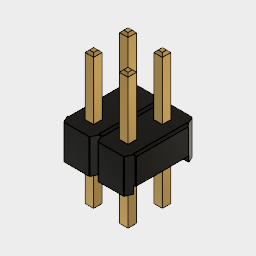
Pin+Header+2x2+TH+Pitch+2 (Autodesk Fusion 360 design; units mm, degrees)
Autodesk Fusion 360 part; units mm, degrees
note: some values were not read from the file. Chosen so that the rebuilt part matches the saved one: which bodies a step acts on; which face or edge a step refers to. Set by a fixed rule: which sketch regions a step uses.
sketch "Sketch1" plane through (0, 0, 0) normal (0, 0, 1) x (1, 0, 0) in component "pins"
  line L0 (0.3175, -0.9525) -> (-0.3175, -0.9525)
  line L1 (-0.3175, -0.9525) -> (-0.3175, -1.5875)
  line L2 (-0.3175, -1.5875) -> (0.3175, -1.5875)
  line L3 (0.3175, -1.5875) -> (0.3175, -0.9525)
  line L4 (0.3175, -0.9525) -> (-0.3175, -1.5875) construction
  line L5 (-0.3175, -0.9525) -> (0.3175, -1.5875) construction
  line L6 (0, 0) -> (0, -2.54) construction
  point P0 (0, -1.27)
  dimension "d8" = 0.635
  dimension "d9" = 0.635
  dimension "d86" = 2.54
  dimension "d88" = 1.27
  measures "d8" distance of L1.end L2.end
  measures "d9" distance of L0.end L1.end
  measures "d86" distance of L6.start L6.end
  measures "d88" distance of P0 L6.end
extrude "Extrude1" add sketch "Sketch1" along normal blind 7 and the other way blind 3 makes body 1 in component "pins"
chamfer "Chamfer1" distance 0.1588 angle 45 8 edges at (0, -1.5875, 7) (0.3175, -1.27, 7) (0, -0.9525, 7) (-0.3175, -1.27, 7) (0.3175, -1.27, -3) (0, -1.5875, -3) (-0.3175, -1.27, -3) (0, -0.9525, -3) on bodies 1 in component "pins"
sketch "Sketch1 (2)" plane through (0, 0, 0) normal (0, 0, 1) x (1, 0, 0) in component "Component"
  line L0 (3.81, -2.54) -> (-1.27, -2.54)
  line L1 (-1.27, -2.54) -> (-1.27, 2.54)
  line L2 (-1.27, 2.54) -> (3.81, 2.54)
  line L3 (3.81, 2.54) -> (3.81, -2.54)
  line L4 (0, 0) -> (-1.27, 0) construction
  line L5 (0, 0) -> (0, 2.54) construction
  line L6 (-1.2247, -1.965) -> (-0.97, -2.5111)
  arc A0 (-0.97, -2.5111) -> (-0.9247, -2.54) centre (-0.9247, -2.49) ccw
  arc A1 (-1.2247, -1.965) -> (-1.27, -1.9361) centre (-1.27, -1.9861) ccw
  arc A2 (1.27, -1.9361) -> (1.2247, -1.965) centre (1.27, -1.9861) ccw
  line L7 (1.2247, -1.965) -> (0.97, -2.5111)
  arc A3 (0.9247, -2.54) -> (0.97, -2.5111) centre (0.9247, -2.49) ccw
  arc A4 (-1.27, 1.9361) -> (-1.2247, 1.965) centre (-1.27, 1.9861) ccw
  arc A5 (-0.9247, 2.54) -> (-0.97, 2.5111) centre (-0.9247, 2.49) ccw
  line L8 (-1.2247, 1.965) -> (-0.97, 2.5111)
  arc A6 (1.2247, 1.965) -> (1.27, 1.9361) centre (1.27, 1.9861) ccw
  arc A7 (0.97, 2.5111) -> (0.9247, 2.54) centre (0.9247, 2.49) ccw
  line L9 (1.2247, 1.965) -> (0.97, 2.5111)
  arc A8 (1.27, 1.9361) -> (1.3153, 1.965) centre (1.27, 1.9861) ccw
  line L10 (1.3153, 1.965) -> (1.57, 2.5111)
  arc A9 (1.6153, 2.54) -> (1.57, 2.5111) centre (1.6153, 2.49) ccw
  arc A10 (3.7647, 1.965) -> (3.81, 1.9361) centre (3.81, 1.9861) ccw
  arc A11 (3.51, 2.5111) -> (3.4647, 2.54) centre (3.4647, 2.49) ccw
  line L11 (3.7647, 1.965) -> (3.51, 2.5111)
  arc A12 (3.81, -1.9361) -> (3.7647, -1.965) centre (3.81, -1.9861) ccw
  arc A13 (3.4647, -2.54) -> (3.51, -2.5111) centre (3.4647, -2.49) ccw
  line L12 (3.7647, -1.965) -> (3.51, -2.5111)
  arc A14 (1.3153, -1.965) -> (1.27, -1.9361) centre (1.27, -1.9861) ccw
  arc A15 (1.57, -2.5111) -> (1.6153, -2.54) centre (1.6153, -2.49) ccw
  line L13 (1.3153, -1.965) -> (1.57, -2.5111)
  dimension "d30" = 5.08
  dimension "d31" = 5.08
  dimension "d40" = 25
  dimension "d41" = 0.05
  dimension "d42" = 0.3
  dimension "d63" = 1.27
  dimension "d66" = 2.54
  dimension "d67" = 0
  measures "d30" distance of L1.end L2.end
  measures "d31" distance of L0.end L1.end
  measures "d40" angle of L1 L6
  measures "d41" radius of A0
  measures "d42" distance of L1 L6.end
  measures "d63" distance of L1 L5
extrude "Extrude1'" add sketch "Sketch1 (2)" along normal blind 2.54 separate body contours L0 L1 L2 L3 L6 A0 A1 A2 L7 A3 A4 A5 L8 A6 A7 L9 A8 L10 A9 A10 A11 L11 A12 A13 L12 A14 A15 L13 makes body 2 in component "Component"
sketch "Sketch3" plane through (0, 0, 0) normal (0, 0, 1) x (1, 0, 0) in component "Component"
  line L0 (-1.27, 2.04) -> (3.81, 2.04)
  line L1 (3.81, 2.04) -> (3.81, -2.04)
  line L2 (3.81, -2.04) -> (-1.27, -2.04)
  line L3 (-1.27, -2.04) -> (-1.27, 2.04)
  line L4 (-1.27, 0) -> (0, 0)
  line L5 (3.81, -2.54) -> (-1.27, -2.54)
  dimension "d68" = 1.27
  dimension "d69" = 5.08
  dimension "d74" = 0.5
  measures "d68" distance of L4.end L3
  measures "d69" distance of L1 L3
  measures "d74" distance of L2 L5
extrude "Extrude4" cut sketch "Sketch3" along normal blind 0.5 bodies 2 in component "Component"
sketch "Sketch2" plane through (0, 0, 2.54) normal (0, 0, 1) x (-1, 0, 0) in component "Component"
  arc A0 (-1.2247, -1.965) -> (-1.3153, -1.965) centre (-1.27, -1.9861) ccw
  line L0 (-1.2247, -1.965) -> (-0.97, -2.5111)
  arc A1 (-0.97, -2.5111) -> (-0.9247, -2.54) centre (-0.9247, -2.49) ccw
  line L1 (-0.9247, -2.54) -> (0.9247, -2.54)
  arc A2 (0.9247, -2.54) -> (0.97, -2.5111) centre (0.9247, -2.49) ccw
  line L2 (0.97, -2.5111) -> (1.2247, -1.965)
  arc A3 (1.27, -1.9361) -> (1.2247, -1.965) centre (1.27, -1.9861) ccw
  line L3 (1.27, -1.9361) -> (1.27, 1.9361)
  arc A4 (1.2247, 1.965) -> (1.27, 1.9361) centre (1.27, 1.9861) ccw
  line L4 (1.2247, 1.965) -> (0.97, 2.5111)
  arc A5 (0.97, 2.5111) -> (0.9247, 2.54) centre (0.9247, 2.49) ccw
  line L5 (0.9247, 2.54) -> (-0.9247, 2.54)
  arc A6 (-0.9247, 2.54) -> (-0.97, 2.5111) centre (-0.9247, 2.49) ccw
  line L6 (-0.97, 2.5111) -> (-1.2247, 1.965)
  arc A7 (-1.3153, 1.965) -> (-1.2247, 1.965) centre (-1.27, 1.9861) ccw
  line L7 (-3.81, 1.9361) -> (-3.81, -1.9361)
  line L8 (-0.3175, 1.5875) -> (0.3175, 1.5875)
  line L9 (0.3175, 1.5875) -> (0.3175, 0.9525)
  line L10 (0.3175, 0.9525) -> (-0.3175, 0.9525)
  line L11 (-0.3175, 0.9525) -> (-0.3175, 1.5875)
  line L12 (-0.3175, 1.5875) -> (0.3175, 0.9525) construction
  line L13 (0.3175, 1.5875) -> (-0.3175, 0.9525) construction
  line L14 (-1.3153, 1.965) -> (-1.57, 2.5111)
  arc A8 (-1.57, 2.5111) -> (-1.6153, 2.54) centre (-1.6153, 2.49) ccw
  line L15 (-1.6153, 2.54) -> (-3.4647, 2.54)
  arc A9 (-3.4647, 2.54) -> (-3.51, 2.5111) centre (-3.4647, 2.49) ccw
  line L16 (-3.51, 2.5111) -> (-3.7647, 1.965)
  arc A10 (-3.81, 1.9361) -> (-3.7647, 1.965) centre (-3.81, 1.9861) ccw
  arc A11 (-3.7647, -1.965) -> (-3.81, -1.9361) centre (-3.81, -1.9861) ccw
  line L17 (-3.7647, -1.965) -> (-3.51, -2.5111)
  arc A12 (-3.51, -2.5111) -> (-3.4647, -2.54) centre (-3.4647, -2.49) ccw
  line L18 (-3.4647, -2.54) -> (-1.6153, -2.54)
  arc A13 (-1.6153, -2.54) -> (-1.57, -2.5111) centre (-1.6153, -2.49) ccw
  line L19 (-1.57, -2.5111) -> (-1.3153, -1.965)
  point P0 (0, 1.27)
  dimension "d47" = 0.635
  dimension "d48" = 0.635
  dimension "d57" = 1.27
  measures "d47" distance of L8.end L9.end
  measures "d48" distance of L9.end L10.end
  measures "d57" distance of L5 P0
extrude "Extrude3" cut sketch "Sketch2" against normal through all contours L8 L9 L10 L11 bodies 2 in component "Component"
pattern_linear "R-Pattern1" count 2 spacing 2.54 along (0, 1, 0) count 2 spacing 2.54 along (1, 0, 0) of "Extrude3" in component "Component"
sketch "Sketch4" plane through (0, 0, 0) normal (0, 1, 0) x (1, 0, 0) in component "Component"
  line L0 (-1.42, -2.54) -> (-1.27, -2.39)
  line L1 (-1.27, -2.39) -> (-1.12, -2.54)
  line L2 (-1.12, -2.54) -> (-1.42, -2.54)
  line L3 (-1.27, -2.39) -> (-1.27, -2.54) construction
  dimension "d75" = 2.54
  dimension "d76" = 1.27
  dimension "d77" = 0.15
  measures "d75" distance of origin L2
  measures "d76" distance of origin L3
  measures "d77" distance of L0.end L3.end
extrude "Extrude5" cut sketch "Sketch4" along normal mid plane 3.9933 bodies 2 in component "Component"
pattern_linear "R-Pattern3" count 3 spacing 2.54 along (1, 0, 0) of "Extrude5" in component "Component"
pattern_linear "R-Pattern1'" count 2 spacing 2.54 along (0, 1, 0) count 2 spacing 2.54 along (1, 0, 0) of bodies 1 makes body 3 at (-0.1058, 0.9525, 0.3862) makes body 4 at (2.8575, -1.3758, 0.3862) makes body 5 at (2.8575, 1.1642, 0.3862) in component "pins"
component "pins" placed x (1, 0, 0) y (0, 1, 0) z (0, 0, 1) at (0, 0, 0)
component "spacers" placed x (1, 0, 0) y (0, 1, 0) z (0, 0, 1) at (0, 0, 0)
component "Component" placed x (1, 0, 0) y (0, 1, 0) z (0, 0, 1) at (0, 0, 0) in component "spacers"
equation "h2x2_pins_wide = 2"
equation "h2x2_pins_deep = 2"
equation "d8 = h2x2_pin_size"
equation "d9 = h2x2_pin_size"
equation "d10 = h2x2_pin_height - h2x2_pin_descent"
equation "d12 = h2x2_pin_descent"
equation "h2x2_spacing = 0.1 in"
equation "d30 = h2x2_spacing * h2x2_pins_wide"
equation "d31 = h2x2_spacing * h2x2_pins_deep"
equation "h2x2_pin_size = 0.025 in"
equation "h2x2_pin_height = 10 mm"
equation "h2x2_pin_descent = 3 mm"
equation "h2x2_spacer_leg_size = 0.5 mm"
equation "h2x2_spacer_leg_height = 0.5 mm"
equation "h2x2_spacer_height = 0.1 in"
equation "h2x2_spacer_taper = 25 deg"
equation "d40 = h2x2_spacer_taper"
equation "d43 = h2x2_spacer_height"
equation "d47 = h2x2_pin_size"
equation "d48 = h2x2_pin_size"
equation "d53 = h2x2_pins_deep"
equation "d54 = h2x2_pins_wide"
equation "d55 = h2x2_spacing"
equation "d56 = h2x2_spacing"
equation "d57 = h2x2_spacing / 2"
equation "d63 = h2x2_spacing / 2"
equation "d64 = h2x2_pins_wide"
equation "d66 = h2x2_spacing"
equation "d68 = h2x2_spacing / 2"
equation "d69 = h2x2_spacing * h2x2_pins_wide"
equation "d72 = h2x2_spacer_leg_height"
equation "d74 = h2x2_spacer_leg_size"
equation "d75 = h2x2_spacer_height"
equation "d76 = h2x2_spacing / 2"
equation "d77 = h2x2_spacer_break_depth"
equation "d78 = h2x2_spacing * h2x2_pins_deep - 2 * ( d42 / tan(h2x2_spacer_taper) - 2 * d41 )"
equation "d80 = h2x2_pins_wide + 1"
equation "d82 = h2x2_spacing"
equation "h2x2_spacer_break_depth = 0.15 mm"
equation "d86 = h2x2_pins_deep * h2x2_spacing / 2"
equation "d88 = h2x2_spacing / 2"
equation "d89 = h2x2_pins_deep"
equation "d90 = h2x2_pins_wide"
equation "d91 = h2x2_spacing"
equation "d92 = h2x2_spacing"
